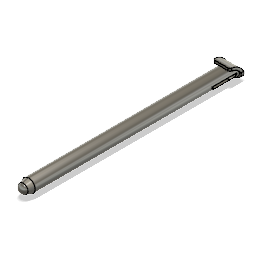
New Nintendo 3DS XL Stylus v5 (Autodesk Fusion 360 design; units mm, degrees)
Autodesk Fusion 360 part; units mm, degrees
note: some values were not read from the file. Chosen so that the rebuilt part matches the saved one: which face or edge a step refers to. Set by a fixed rule: which sketch regions a step uses.
sketch "Sketch1" plane through (0, 0, 0) normal (0, 0, 1) x (1, 0, 0)
  circle A0 centre (0, 0) radius 2.6
  dimension "d1" = 5.2
  constraint coincident A0.centre origin
  measures "d1" diameter of A0
extrude "Extrude1" add sketch "Sketch1" along normal blind 86
sketch "Sketch2" plane through (0, 0, 0) normal (1, 0, 0) x (0, 0, -1)
  line L0 (0, 0) -> (0, -2.7)
  line L1 (0, -2.7) -> (0, -3.4)
  line L2 (0, -3.4) -> (-1, -3.4)
  line L3 (0, 0) -> (-6, 0)
  line L4 (-6, 0) -> (-6, 3.5)
  line L5 (-6, 3.5) -> (-6, 2.5)
  line L6 (-6, 2.5) -> (-7, 2.5)
  line L7 (-6, 3.5) -> (-7, 3.5)
  arc A0 (0, -3.4) -> (-6, 3.5) centre (-6, -2.5587) ccw
  circle A1 centre (-6, -2.5587) radius 5.0587
  line L8 (0, -2.7) -> (-0.05, -2.7)
  line L9 (-0.05, -2.7) -> (-0.9433, -2.7)
  line L10 (-0.9433, -2.7) -> (-0.9433, -3.4)
  line L11 (-6, 3.5) -> (0, 3.5)
  line L12 (0, 3.5) -> (0, -3.4)
  line L13 (0, -3.4) -> (-6, -3.4)
  line L14 (-6, -3.4) -> (-6, 3.5)
  dimension "d4" = 2.7
  dimension "d5" = 0.7
  dimension "d6" = 1
  dimension "d7" = 6
  dimension "d8" = 3.5
  dimension "d9" = 1
  dimension "d10" = 1
  dimension "d11" = 1
  constraint coincident L0.start L3.start
  constraint vertical L0
  constraint parallel L0 L1
  constraint perpendicular L1 L2
  constraint perpendicular L0 L3
  constraint perpendicular L3 L4
  constraint parallel L4 L5
  constraint perpendicular L4 L6
  constraint perpendicular L5 L7
  constraint tangent L7 A0
  constraint concentric A0 A1
  constraint coincident L5.end A1
  constraint perpendicular L1 L8
  constraint coincident A1 L9.end
  constraint perpendicular L1 L9
  constraint coincident L2 L10.end
  constraint perpendicular L2 L10
  constraint horizontal L11
  constraint vertical L12
  constraint horizontal L13
  constraint vertical L14
  measures "d4" distance of L0.start L0.end
  measures "d5" distance of L0.end L1.end
  measures "d6" distance of L1.end L2.end
  measures "d7" distance of L0.start L3.end
  measures "d8" distance of L3.end L4.end
  measures "d9" distance of L4.end L5.end
  measures "d10" distance of L5.end L6.end
  measures "d11" distance of L4.end L7.end
extrude "Extrude2" cut sketch "Sketch2" along normal blind -14.5 and the other way blind -14 contours L0 L3 A0 L12 | L3 A0 L11 L12
extrude "Extrude3" add sketch "Sketch2" along normal blind 3.45 and the other way blind 3.45 contours L0 L3 A0 A1 L8 L9 L12 | L3 L4 L5 A0 A1 L14 | L1 L2 L8 L9 L10 L12 L13
sketch "Sketch3" plane through (0, 0, 0) normal (0, 0, 1) x (1, 0, 0)
  circle A0 centre (0, 0) radius 3.4
  line L0 (0, 0) -> (-4.7, 0)
  line L1 (-4.7, 0) -> (4.4, 0)
  line L2 (4.4, 0) -> (4.4, -3.4)
  line L3 (4.4, -3.4) -> (-4.7, -3.4)
  line L4 (-4.7, -3.4) -> (-4.7, 0)
  dimension "d20" = 9.1
  constraint coincident A0.centre L0.start
  constraint horizontal L0
  constraint horizontal L1
  constraint vertical L2
  constraint horizontal L3
  constraint vertical L4
  measures "d20" distance of L0.end L1.end
extrude "Extrude4" cut sketch "Sketch3" along normal blind 2.8 contours A0 L1 L2 L3 | A0 L0 L1 L3 L4
fillet "Fillet1" radius 0.75 2 edges at (-3.45, 3, 6) (3.45, 3, 6)
move_face "MoveFace1" by (0.05, 0, 0) 1 faces at (-3.45, 0.2545, 1.0259)
move_face "MoveFace2" by (-0.05, 0, 0) 1 faces at (3.45, 0.2545, 1.0259)
sketch "Sketch4" plane through (0, 0, 0) normal (1, 0, 0) x (0, 0, -1)
  line L0 (0, 0) -> (-8.6, 0)
  line L1 (-8.6, 0) -> (-8.6, -2.7)
  line L2 (-8.6, -2.7) -> (-6.1, -2.7)
  ellipse E0 centre (-7.35, -2.7) end of major axis (-6.1, -2.7) minor radius 0.5
  line L3 (-8.6, -2.7) -> (-6.1, -2.7) construction
  line L4 (-7.35, -3.2) -> (-7.35, -2.2) construction
  line L5 (-7.35, -2.7) -> (-7.35, 0)
  line L6 (-7.35, 0) -> (-4.35, 0)
  line L7 (-7.35, 0) -> (-10.35, 0)
  line L8 (-4.35, 1.95) -> (-10.35, 1.95)
  arc A0 (-10.35, 1.95) -> (-10.35, -1.95) centre (-10.35, 0) ccw
  line L9 (-10.35, -1.95) -> (-4.35, -1.95)
  arc A1 (-4.35, -1.95) -> (-4.35, 1.95) centre (-4.35, 0) ccw
  line L10 (-4.35, 0) -> (-10.35, 0) construction
  line L11 (-10.35, 0) -> (-12.3, 0)
  line L12 (-7.35, -2.7) -> (-6.45, -2.7)
  ellipse E1 centre (-7.35, -2.7) end of major axis (-6.1, -2.7) minor radius 0.75
  line L13 (-8.6, -2.7) -> (-6.1, -2.7) construction
  line L14 (-7.35, -3.45) -> (-7.35, -1.95) construction
  dimension "d27" = 8.6
  dimension "d28" = 2.7
  dimension "d29" = 2.5
  dimension "d30" = 1
  dimension "d31" = 3
  dimension "d32" = 3
  dimension "d33" = 3.9
  dimension "d44" = 0.9
  dimension "d45" = 1.5
  constraint coincident L0.start origin
  constraint horizontal L0
  constraint perpendicular L0 L1
  constraint perpendicular L1 L2
  constraint midpoint L2 E0.centre
  constraint parallel L2 L3
  constraint coincident L1.end E0
  constraint coincident E0 L4.start
  constraint coincident E0 L4.end
  constraint coincident E0.centre L5.start
  constraint coincident L0 L5.end
  constraint perpendicular L0 L5
  constraint perpendicular L5 L6
  constraint perpendicular L1 L7
  constraint tangent L8 A0
  constraint tangent A0 L9
  constraint parallel L8 L9
  constraint tangent L9 A1
  constraint tangent L8 A1
  constraint coincident L7.end A0.centre
  constraint perpendicular L5 L10
  constraint coincident L6.end A1.centre
  constraint midpoint A0 L11.end
  constraint parallel L2 L12
  constraint coincident L1.end E1
  constraint coincident E1 L14.start
  constraint coincident E1 L14.end
  measures "d27" distance of L0.start L0.end
  measures "d28" distance of L0.end L1.end
  measures "d29" distance of L1.end L2.end
  measures "d31" distance of L5.end L6.end
  measures "d32" distance of L5.end L7.end
  measures "d33" diameter of A0
  measures "d44" distance of E0.centre L12.end
extrude "Extrude5" cut sketch "Sketch4" along normal mid plane 10 contours L0 L5 L6 L9 A1 | L0 L1 L5 L7 L9 | L1 L7 A0 L9 L11
extrude "Extrude6" add sketch "Sketch4" along normal mid plane 0.75 contours L2 E0 L5 | L2 E0 L5 L12 | L2 E0 L12
sketch "Sketch5" plane through (0, 0, 86) normal (0, 0, 1) x (1, 0, 0)
  circle A0 centre (0, 0) radius 2.6
  circle A1 centre (0, 0) radius 1.5
  circle A2 centre (0, 0) radius 2.7
  constraint concentric A0 A1
  constraint coincident A0.centre A1.centre
extrude "Extrude7" cut sketch "Sketch5" against normal blind 3.6 contours A0 | A2
chamfer "Chamfer1" distance 3.6 distance2 1.1 1 edges at (-1.3985, -0.5424, 82.4) measured on face at (1.4981, -0.0748, 83.6)
fillet "Fillet3" radius 2 2 edges at (-1.5, 0, 85.9993) (-1.5, 0, 86)
moveface "MoveFace3" [suppressed]
extrude "Extrude8" [suppressed]
equation "d4 = ( 5.4 / 2 ) * 1 mm"
equation "d8 = ( ( 5.4 / 2 ) * 1 mm ) + 0.8 mm"
equation "d16 = ( 6.9 / 2 ) * 1 mm"
equation "d18 = ( 6.9 / 2 ) * 1 mm"
equation "d28 = ( 5.4 / 2 ) * 1 mm"
equation "d33 = 4.400 mm - 0.5 mm"
equation "d36 = 0.75 mm / 2"
equation "d38 = ( -1.2 * 3 ) * 1 mm"
named bodies: "New 3DS XL Stylus"
